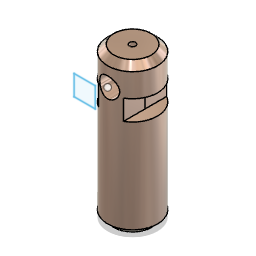
Cu tube milled v2 (Autodesk Fusion 360 design; units mm, degrees)
Autodesk Fusion 360 part; units mm, degrees
cylinder "CylinderPrimitive1" add diameter 2 height 6 placed x (1, 0, 0) y (0, 0, -1) z (0, 1, 0) at (0, 0, 0)
hole "Hole1" at (0, 0, 0) direction (0, 1, 0) diameter 1 depth 4.5 tip angle 118
hole "Hole2" at (0, 0, 0) direction (0, 1, 0) diameter 0.25 depth 12.5 tip angle 118
chamfer "Chamfer1" distance 0.25 angle 45 2 edges at (-0.9323, 6, 0.3616) (-0.9323, 0, -0.3616) measured on face at (0.7045, 6, 0.0528) measured on face at (0.8291, 0, 0.0621)
ref_plane "WorkPlane1" through (0, 3, 1) normal (0, 0, 1) x (1, 0, 0)
sketch "Sketch2" plane through (0, 3, 1) normal (0, 0, 1) x (1, 0, 0)
  line L0 (-1.3486, 1.8087) -> (-0.5, 1.8087)
  line L1 (-0.5, 1.8087) -> (-0.5, 1)
  line L2 (-0.5, 1) -> (-1.3486, 1)
  line L3 (-1.3486, 1) -> (-1.3486, 1.8087)
  point P0 (0, 2)
  constraint horizontal L0
  constraint vertical L1
  constraint horizontal L2
  constraint vertical L3
hole "Hole3" at (0, 5, 1) direction (0, 0, -1) diameter 0.8 depth 0.7 tip angle 180
extrude "Extrude1" cut sketch "Sketch2" against normal blind 2.5
mirror "Mirror1" about plane through (0, 0, 0) normal (1, 0, 0) of "Extrude1"
